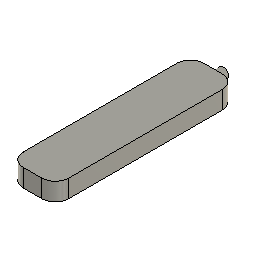
Nova-Q (Autodesk Fusion 360 archive; units mm, degrees)
design "Hub"
Autodesk Fusion 360 part; units mm, degrees
sketch "Sketch1" plane through (0, 0, 0) normal (0, 0, 1) x (1, 0, 0)
  line L0 (6.1, 60.05) -> (-6.1, 60.05)
  line L1 (-15.1, 51.05) -> (-15.1, -51.05)
  line L2 (-6.1, -60.05) -> (6.1, -60.05)
  line L3 (15.1, -51.05) -> (15.1, 51.05)
  line L4 (15.1, 60.05) -> (-15.1, -60.05) construction
  line L5 (-15.1, 60.05) -> (15.1, -60.05) construction
  arc A0 (-6.1, 60.05) -> (-15.1, 51.05) centre (-6.1, 51.05) ccw
  arc A1 (15.1, 51.05) -> (6.1, 60.05) centre (6.1, 51.05) ccw
  arc A2 (6.1, -60.05) -> (15.1, -51.05) centre (6.1, -51.05) ccw
  arc A3 (-15.1, -51.05) -> (-6.1, -60.05) centre (-6.1, -51.05) ccw
  dimension "d1" = 30.2
  dimension "d2" = 120.1
  dimension "d3" = 9
  constraint horizontal L0
  constraint perpendicular L0 L1
  constraint parallel L0 L2
  constraint parallel L1 L3
  constraint coincident L4 origin
  constraint coincident L5 origin
  constraint coincident L5.start L0
  constraint coincident L5.start L1
  constraint tangent L0 A0
  constraint tangent L1 A0
  constraint coincident L4.start L0
  constraint coincident L4.start L3
  constraint tangent L0 A1
  constraint tangent L3 A1
  constraint equal A0 A1
  constraint coincident L5.end L3
  constraint coincident L5.end L2
  constraint tangent L3 A2
  constraint tangent L2 A2
  constraint equal A0 A2
  constraint coincident L4.end L1
  constraint coincident L4.end L2
  constraint tangent L1 A3
  constraint tangent L2 A3
  constraint equal A0 A3
  measures "d1" distance of L4.end L5.end
  measures "d2" distance of L5.start L4.end
  measures "d3" radius of A0
extrude "Extrude1" add sketch "Sketch1" along normal blind 11.9
sketch "Sketch2" plane through (0, 60.05, 0) normal (0, 1, 0) x (-1, 0, 0)
  line L0 (-6.1, 0) -> (6.1, 0)
  line L1 (6.1, 0) -> (6.1, 11.9)
  line L2 (6.1, 11.9) -> (-6.1, 11.9)
  line L3 (-6.1, 11.9) -> (-6.1, 0)
  line L4 (0, 11.9) -> (0, 0) construction
  circle A0 centre (0, 5.95) radius 3.425
  dimension "d6" = 6.85
  constraint midpoint L2 L4.start
  constraint coincident L4.end origin
  constraint midpoint L4 A0.centre
  measures "d6" diameter of A0
extrude "Extrude2" add sketch "Sketch2" along normal blind 6.9 contours A0

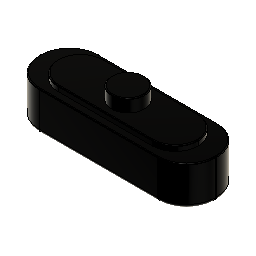
design "Camera"
Autodesk Fusion 360 part; units mm, degrees
sketch "Sketch1" plane through (0, 0, 0) normal (0, 0, 1) x (1, 0, 0)
  line L0 (30.6, 15.36) -> (-30.6, 15.36)
  line L1 (-45.6, 0.36) -> (-45.6, -0.36)
  line L2 (-30.6, -15.36) -> (30.6, -15.36)
  line L3 (45.6, -0.36) -> (45.6, 0.36)
  line L4 (45.6, 15.36) -> (-45.6, -15.36) construction
  line L5 (-45.6, 15.36) -> (45.6, -15.36) construction
  arc A0 (-30.6, 15.36) -> (-45.6, 0.36) centre (-30.6, 0.36) ccw
  arc A1 (-45.6, -0.36) -> (-30.6, -15.36) centre (-30.6, -0.36) ccw
  arc A2 (30.6, -15.36) -> (45.6, -0.36) centre (30.6, -0.36) ccw
  arc A3 (45.6, 0.36) -> (30.6, 15.36) centre (30.6, 0.36) ccw
  dimension "d1" = 91.2
  dimension "d2" = 30.72
  dimension "d3" = 15
  constraint horizontal L0
  constraint perpendicular L0 L1
  constraint parallel L0 L2
  constraint parallel L1 L3
  constraint coincident L4 origin
  constraint coincident L5 origin
  constraint coincident L5.start L0
  constraint coincident L5.start L1
  constraint tangent L0 A0
  constraint tangent L1 A0
  constraint coincident L4.end L1
  constraint coincident L4.end L2
  constraint tangent L1 A1
  constraint tangent L2 A1
  constraint equal A0 A1
  constraint coincident L5.end L2
  constraint coincident L5.end L3
  constraint tangent L2 A2
  constraint tangent L3 A2
  constraint equal A0 A2
  constraint coincident L4.start L0
  constraint coincident L4.start L3
  constraint tangent L0 A3
  constraint tangent L3 A3
  constraint equal A0 A3
  measures "d1" distance of L4.end L5.end
  measures "d2" distance of L5.start L4.end
  measures "d3" radius of A0
extrude "Extrude1" add sketch "Sketch1" along normal blind 20.2
sketch "Sketch2" plane through (0, 0, 20.2) normal (0, 0, 1) x (-1, 0, 0)
  arc A0 (-45.6, -0.36) -> (-30.6, -15.36) centre (-30.6, -0.36) ccw
  line L0 (-30.6, -15.36) -> (30.6, -15.36)
  arc A1 (30.6, -15.36) -> (45.6, -0.36) centre (30.6, -0.36) ccw
  line L1 (45.6, -0.36) -> (45.6, 0.36)
  arc A2 (45.6, 0.36) -> (30.6, 15.36) centre (30.6, 0.36) ccw
  line L2 (30.6, 15.36) -> (-30.6, 15.36)
  arc A3 (-30.6, 15.36) -> (-45.6, 0.36) centre (-30.6, 0.36) ccw
  line L3 (-45.6, 0.36) -> (-45.6, -0.36)
  line L4 (-24.3, -11.8) -> (24.3, -11.8)
  line L5 (36.3, 0.2) -> (36.3, -0.2)
  line L6 (24.3, 11.8) -> (-24.3, 11.8)
  line L7 (-36.3, -0.2) -> (-36.3, 0.2)
  line L8 (-36.3, -11.8) -> (36.3, 11.8) construction
  line L9 (36.3, -11.8) -> (-36.3, 11.8) construction
  arc A4 (24.3, -11.8) -> (36.3, 0.2) centre (24.3, 0.2) ccw
  arc A5 (36.3, -0.2) -> (24.3, 11.8) centre (24.3, -0.2) ccw
  arc A6 (-24.3, 11.8) -> (-36.3, -0.2) centre (-24.3, -0.2) ccw
  arc A7 (-36.3, 0.2) -> (-24.3, -11.8) centre (-24.3, 0.2) ccw
  dimension "d6" = 72.6
  dimension "d7" = 23.6
  dimension "d8" = 12
  constraint horizontal L4
  constraint perpendicular L4 L5
  constraint parallel L4 L6
  constraint parallel L5 L7
  constraint coincident L8 origin
  constraint coincident L9 origin
  constraint coincident L9.start L4
  constraint coincident L9.start L5
  constraint tangent L4 A4
  constraint tangent L5 A4
  constraint coincident L8.end L5
  constraint coincident L8.end L6
  constraint tangent L5 A5
  constraint tangent L6 A5
  constraint equal A4 A5
  constraint coincident L9.end L6
  constraint coincident L9.end L7
  constraint tangent L6 A6
  constraint tangent L7 A6
  constraint equal A4 A6
  constraint coincident L8.start L7
  constraint coincident L8.start L4
  constraint tangent L7 A7
  constraint tangent L4 A7
  constraint equal A4 A7
  measures "d6" distance of L8.end L9.end
  measures "d7" distance of L9.start L8.end
  measures "d8" radius of A4
extrude "Extrude2" add sketch "Sketch2" along normal blind 2.7 contours L4 L6 A4 A5 A6 A7
sketch "Sketch3" plane through (0, 0, 22.9) normal (0, 0, 1) x (-1, 0, 0)
  arc A0 (-24.3, 11.8) -> (-36.2983, 0) centre (-24.3, -0.2) ccw
  arc A1 (-36.2983, 0) -> (-24.3, -11.8) centre (-24.3, 0.2) ccw
  line L0 (-24.3, -11.8) -> (24.3, -11.8)
  arc A2 (24.3, -11.8) -> (36.2983, 0) centre (24.3, 0.2) ccw
  arc A3 (36.2983, 0) -> (24.3, 11.8) centre (24.3, -0.2) ccw
  line L1 (24.3, 11.8) -> (-24.3, 11.8)
  circle A4 centre (0, 0) radius 8.5
  dimension "d11" = 17
  constraint coincident A4.centre origin
  measures "d11" diameter of A4
extrude "Extrude3" add sketch "Sketch3" along normal blind 6.5 contours A4
fillet "Fillet1" radius 2 8 edges at (-41.2066, 10.9666, 0) (-45.6, 0, 0) (-41.2066, -10.9666, 0) (0, -15.36, 0) (41.2066, -10.9666, 0) (45.6, 0, 0) (41.2066, 10.9666, 0) (0, 15.36, 0)
fillet "Fillet2" radius 0.5 8 edges at (-41.2066, 10.9666, 20.2) (-45.6, 0, 20.2) (-41.2066, -10.9666, 20.2) (0, -15.36, 20.2) (41.2066, -10.9666, 20.2) (45.6, 0, 20.2) (41.2066, 10.9666, 20.2) (0, 15.36, 20.2)
fillet "Fillet3" radius 0.5 6 edges at (32.7143, 8.3557, 22.9) (0, 11.8, 22.9) (-32.7143, 8.3557, 22.9) (-32.7143, -8.3557, 22.9) (0, -11.8, 22.9) (32.7143, -8.3557, 22.9)
fillet "Fillet4" radius 0.5 1 edges at (7.9248, 3.0737, 29.4)
sketch "Sketch4" plane through (0, 0, 0) normal (0, 0, -1) x (1, 0, 0)
  arc A0 (-43.6, -0.36) -> (-30.6, -13.36) centre (-30.6, -0.36) ccw
  line L0 (-30.6, -13.36) -> (30.6, -13.36)
  arc A1 (30.6, -13.36) -> (43.6, -0.36) centre (30.6, -0.36) ccw
  line L1 (43.6, -0.36) -> (43.6, 0.36)
  arc A2 (43.6, 0.36) -> (30.6, 13.36) centre (30.6, 0.36) ccw
  line L2 (30.6, 13.36) -> (-30.6, 13.36)
  arc A3 (-30.6, 13.36) -> (-43.6, 0.36) centre (-30.6, 0.36) ccw
  line L3 (-43.6, 0.36) -> (-43.6, -0.36)
  line L4 (7.45, 4.55) -> (-7.45, 4.55)
  line L5 (-7.45, 4.55) -> (-7.45, -4.55)
  line L6 (-7.45, -4.55) -> (7.45, -4.55)
  line L7 (7.45, -4.55) -> (7.45, 4.55)
  line L8 (7.45, 4.55) -> (-7.45, -4.55) construction
  line L9 (-7.45, 4.55) -> (7.45, -4.55) construction
  dimension "d22" = 14.9
  dimension "d23" = 9.1
  constraint horizontal L4
  constraint perpendicular L4 L5
  constraint parallel L4 L6
  constraint parallel L5 L7
  constraint coincident L8 origin
  constraint coincident L9 origin
  measures "d22" distance of L5.end L6.end
  measures "d23" distance of L4.end L5.end
extrude "Extrude4" add sketch "Sketch4" along normal blind 9.1 contours L4 L5 L6 L7
sketch "Sketch5" plane through (-7.45, 0, 0) normal (-1, 0, 0) x (0, -1, 0)
  line L0 (4.55, 0) -> (-4.55, 0)
  line L1 (-4.55, 0) -> (-4.55, -9.1)
  line L2 (-4.55, -9.1) -> (4.55, -9.1)
  line L3 (4.55, -9.1) -> (4.55, 0)
  line L4 (4.55, -9.1) -> (-4.55, -9.1)
  line L5 (-4.55, 0) -> (-4.55, -9.1)
  line L6 (4.55, 0) -> (-4.625, 0)
  line L7 (-4.625, 0) -> (-4.625, -3.93)
  line L8 (-0.125, -8.43) -> (0.25, -8.43)
  line L9 (4.55, -3.9351) -> (4.55, 0)
  circle A0 centre (0, -4.55) radius 4.55
  dimension "d27" = 9.1
  constraint horizontal L6
  constraint vertical L7
  constraint horizontal L8
  constraint vertical L9
  constraint coincident L0.start L3.end
  constraint tangent L2 A0
  constraint tangent L5 A0
  measures "d27" diameter of A0
extrude "Extrude5" cut sketch "Sketch5" against normal blind 17.5 contours L2 L3 L4 A0 | L1 L2 L4 L5 A0
sketch "Sketch6" plane through (-7.45, 0, 0) normal (-1, 0, 0) x (0, -1, 0)
  arc A0 (-4.55, -4.55) -> (4.55, -4.55) centre (0, -4.55) ccw
  line L0 (4.55, -4.55) -> (4.55, 0)
  line L1 (4.55, 0) -> (-4.55, 0)
  line L2 (-4.55, 0) -> (-4.55, -4.55)
  circle A1 centre (0, -4.55) radius 1.965
  dimension "d30" = 3.93
  constraint concentric A0 A1
  measures "d30" diameter of A1
extrude "Extrude6" cut sketch "Sketch6" against normal blind 24.5 contours A1

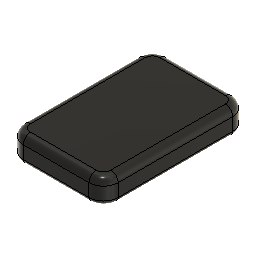
design "Power_bank"
Autodesk Fusion 360 part; units mm, degrees
sketch "Sketch1" plane through (0, 0, 0) normal (0, 0, 1) x (1, 0, 0)
  line L0 (22.5, 49.25) -> (-22.5, 49.25)
  line L1 (-32.5, 39.25) -> (-32.5, -39.25)
  line L2 (-22.5, -49.25) -> (22.5, -49.25)
  line L3 (32.5, -39.25) -> (32.5, 39.25)
  line L4 (32.5, 49.25) -> (-32.5, -49.25) construction
  line L5 (-32.5, 49.25) -> (32.5, -49.25) construction
  arc A0 (-22.5, 49.25) -> (-32.5, 39.25) centre (-22.5, 39.25) ccw
  arc A1 (32.5, 39.25) -> (22.5, 49.25) centre (22.5, 39.25) ccw
  arc A2 (22.5, -49.25) -> (32.5, -39.25) centre (22.5, -39.25) ccw
  arc A3 (-32.5, -39.25) -> (-22.5, -49.25) centre (-22.5, -39.25) ccw
  dimension "d1" = 65
  dimension "d2" = 98.5
  dimension "d3" = 10
  constraint horizontal L0
  constraint perpendicular L0 L1
  constraint parallel L0 L2
  constraint parallel L1 L3
  constraint coincident L4 origin
  constraint coincident L5 origin
  constraint coincident L5.start L0
  constraint coincident L5.start L1
  constraint tangent L0 A0
  constraint tangent L1 A0
  constraint coincident L4.start L0
  constraint coincident L4.start L3
  constraint tangent L0 A1
  constraint tangent L3 A1
  constraint equal A0 A1
  constraint coincident L5.end L3
  constraint coincident L5.end L2
  constraint tangent L3 A2
  constraint tangent L2 A2
  constraint equal A0 A2
  constraint coincident L4.end L2
  constraint coincident L4.end L1
  constraint tangent L2 A3
  constraint tangent L1 A3
  constraint equal A0 A3
  measures "d1" distance of L4.end L5.end
  measures "d2" distance of L5.start L4.end
  measures "d3" radius of A0
extrude "Extrude1" add sketch "Sketch1" along normal blind 16.8
fillet "Fillet1" radius 3 8 edges at (0, 49.25, 0) (-29.5711, 46.3211, 0) (-32.5, 0, 0) (-29.5711, -46.3211, 0) (0, -49.25, 0) (29.5711, -46.3211, 0) (32.5, 0, 0) (29.5711, 46.3211, 0)
fillet "Fillet2" radius 5 8 edges at (29.5711, 46.3211, 16.8) (0, 49.25, 16.8) (-29.5711, 46.3211, 16.8) (-32.5, 0, 16.8) (-29.5711, -46.3211, 16.8) (0, -49.25, 16.8) (29.5711, -46.3211, 16.8) (32.5, 0, 16.8)

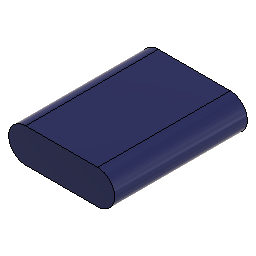
design "Battery 12v"
Autodesk Fusion 360 part; units mm, degrees
sketch "Sketch1" plane through (0, 0, 0) normal (0, 0, 1) x (1, 0, 0)
  line L0 (0, 0) -> (56, 0)
  line L1 (56, 0) -> (56, 70.1)
  line L2 (56, 70.1) -> (0, 70.1)
  line L3 (0, 70.1) -> (0, 0)
  dimension "d1" = 56
  dimension "d2" = 70.1
  constraint horizontal L0
  constraint vertical L1
  constraint horizontal L2
  constraint vertical L3
  constraint coincident L0.start L3.end
  measures "d1" distance of L0.start L0.end
  measures "d2" distance of L0.start L2.end
extrude "Extrude1" add sketch "Sketch1" along normal blind 18
sketch "Sketch2" plane through (0, 0, 0) normal (0, -1, 0) x (1, 0, 0)
  line L0 (0, 0) -> (56, 0)
  line L1 (56, 0) -> (56, 18)
  line L2 (56, 18) -> (0, 18)
  line L3 (0, 18) -> (0, 0)
  line L4 (0, 9) -> (56, 9) construction
  circle A0 centre (9, 9) radius 9
  circle A1 centre (47, 9) radius 9
  circle A2 centre (29, 9) radius 9
  dimension "d5" = 18
  dimension "d6" = 18
  dimension "d7" = 18
  constraint midpoint L3 L4.start
  constraint midpoint L1 L4.end
  constraint coincident L4 A0.centre
  constraint tangent L3 A0
  constraint coincident L4 A1.centre
  constraint tangent L1 A1
  constraint coincident L4 A2.centre
  constraint tangent A1 A2
  measures "d5" diameter of A0
  measures "d6" diameter of A1
  measures "d7" diameter of A2
extrude "Extrude2" cut sketch "Sketch2" against normal blind 96 contours L0 L3 A0 | L2 L3 A0 | L0 L1 A1 | L1 L2 A1
